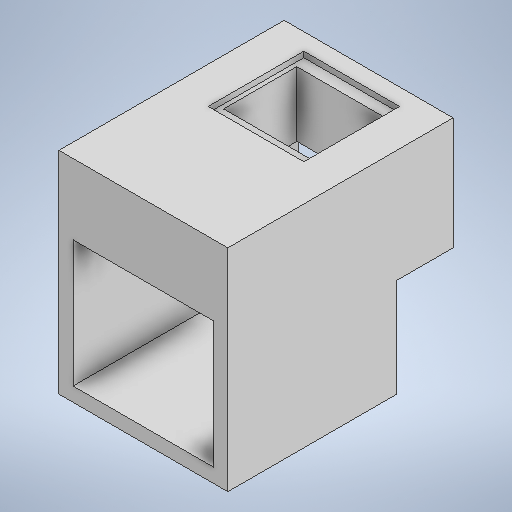
# Autodesk Inventor part: color sensor holder
Saved by Autodesk Inventor 2025.3 (Build 293356000, 356)
## iProperties
Created: 2026-04-15
Part Number: color sensor holder
Material: Generic
Document SubType Name: Modeling
Designer: kamal
Density: 1 g/cm^3
Appearance: Default
Author: kamal
Autodesk Inventor part; units mm, degrees
ref_plane "YZ Plane" through (0, 0, 0) normal (1, 0, 0) x (0, 1, 0)
ref_plane "XZ Plane" through (0, 0, 0) normal (0, 1, 0) x (-1, 0, 0)
ref_plane "XY Plane" through (0, 0, 0) normal (0, 0, 1) x (1, 0, 0)
sketch "Sketch1" plane through (0, 0, 0) normal (0, 0, 1) x (1, 0, 0)
  line L0 (0, 0) -> (0, 50) construction
  line L1 (0, 0) -> (-30, 0)
  line L2 (-30, 0) -> (-30, 55)
  line L3 (-30, 55) -> (0, 55)
  line L4 (0, 55) -> (0, 50) construction
  line L5 (0, 50) -> (-25, 50)
  line L6 (-25, 50) -> (-25, 5)
  line L7 (-25, 5) -> (0, 5)
  line L8 (0, 5) -> (0, 0) construction
  line L9 (0, 0) -> (30, 0)
  line L10 (30, 0) -> (30, 55)
  line L11 (30, 55) -> (0, 55)
  line L12 (0, 50) -> (25, 50)
  line L13 (25, 50) -> (25, 5)
  line L14 (25, 5) -> (0, 5)
  dimension "d0" = 50
  dimension "d1" = 30
  dimension "d2" = 55
  dimension "d3" = 25
  dimension "d4" = 45
  constraints: 30 end point, 4 perpendicular, 4 symmetric about line, 3 horizontal, 2 vertical, 1 point on line
  measures "d0" distance of L0.start L0.end
  measures "d1" distance of L0.start L1.end
  measures "d2" distance of L1.end L2.end
  measures "d3" distance of L0.end L5.end
  measures "d4" distance of L5.end L6.end
extrude "Extrusion1" add sketch "Sketch1" along normal blind 80
sketch "Sketch2" plane through (-30, 55, 0) normal (0, 1, 0) x (1, 0, 0)
  line L0 (13, -6) -> (47, -6)
  line L1 (47, -6) -> (47, -40)
  line L2 (47, -40) -> (13, -40)
  line L3 (13, -40) -> (13, -6)
  line L4 (13, -6) -> (47, -40) construction
  line L5 (47, -6) -> (13, -40) construction
  line L6 (14.5, -10) -> (45.5, -10)
  line L7 (45.5, -10) -> (45.5, -36)
  line L8 (45.5, -36) -> (14.5, -36)
  line L9 (14.5, -36) -> (14.5, -10)
  line L10 (14.5, -10) -> (45.5, -36) construction
  line L11 (45.5, -10) -> (14.5, -36) construction
  line L12 (0, 0) -> (0, -80) projected
  line L13 (60, 0) -> (0, 0) projected
  line L14 (60, -80) -> (0, -80) projected
  line L15 (60, 0) -> (60, -80) projected
  point P0 (30, 0)
  point P1 (30, -23)
  dimension "d7" = 34
  dimension "d8" = 34
  dimension "d9" = 31
  dimension "d10" = 26
  dimension "d11" = 30
  dimension "d12" = 23
  constraints: 24 end point, 4 midpoint, 4 parallel, 2 horizontal, 2 perpendicular
  measures "d7" distance of L2.start L3.start
  measures "d8" distance of L0.end L2.start
  measures "d9" distance of L8.start L9.start
  measures "d10" distance of L6.end L8.start
  measures "d11" distance from line of L12 point (30, -23)
  measures "d12" distance from line of L13 point (30, -23)
extrude "Extrusion2" cut sketch "Sketch2" against normal blind 10 contours L6 L7 L8 L9
extrude "Extrusion3" add sketch "Sketch2" along normal blind 10 contours L0 L1 L2 L3
extrude "Extrusion4" add sketch "Sketch2" along normal blind 20 contours L13 L15 L14 L12
sketch "Sketch3" plane through (-30, 0, 0) normal (-1, 0, 0) x (0, 0, 1)
  line L0 (0, 0) -> (20, 0)
  line L1 (20, 0) -> (20, 35)
  line L2 (20, 35) -> (0, 35)
  line L3 (0, 35) -> (0, 0)
  dimension "d19" = 20
  dimension "d20" = 35
  constraints: 8 end point, 2 parallel, 1 horizontal, 1 perpendicular
  measures "d19" distance of L2.end L1.end
  measures "d20" distance of L0.end L1.end
extrude "Extrusion5" cut sketch "Sketch3" against normal through all
sketch "Sketch4" plane through (-30, 65, 0) normal (0, 1, 0) x (1, 0, 0)
  line L0 (13, -40) -> (47, -40) projected
  line L1 (47, -40) -> (47, -6) projected
  line L2 (47, -6) -> (13, -6) projected
  line L3 (13, -6) -> (13, -40) projected
  line L4 (14.5, -36) -> (14.5, -10) projected
  line L5 (14.5, -10) -> (45.5, -10) projected
  line L6 (45.5, -10) -> (45.5, -36) projected
  line L7 (45.5, -36) -> (14.5, -36) projected
  point P0 (30, 0)
extrude "Extrusion6" add sketch "Sketch4" along normal blind 8
body "Solid1"
